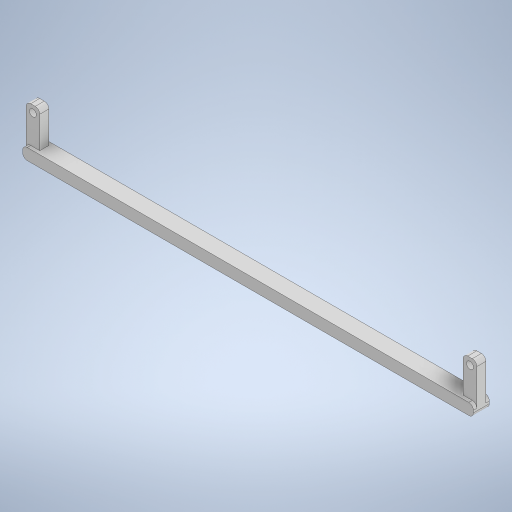
# Autodesk Inventor part: Brace_equal
Saved by Autodesk Inventor 2024.3 (Build 283343000, 343)
## iProperties
Created: 2024-11-11
Part Number: Brace_equal
Material: Generic
Document SubType Name: Modeling
Designer: magn1
Density: 1 g/cm^3
Appearance: Default
Author: magn1
Autodesk Inventor part; units mm, degrees
ref_plane "YZ Plane" through (0, 0, 0) normal (1, 0, 0) x (0, 1, 0)
ref_plane "XZ Plane" through (0, 0, 0) normal (0, 1, 0) x (-1, 0, 0)
ref_plane "XY Plane" through (0, 0, 0) normal (0, 0, 1) x (1, 0, 0)
sketch "Sketch1" plane through (0, 0, 0) normal (0, 1, 0) x (-1, 0, 0)
  line L0 (99.05, 3.5) -> (-99.05, 3.5)
  line L1 (-99.05, 3.5) -> (-99.05, -3.5)
  line L2 (-99.05, -3.5) -> (99.05, -3.5)
  line L3 (99.05, -3.5) -> (99.05, 3.5)
  line L4 (99.05, 3.5) -> (-99.05, -3.5) construction
  line L5 (-99.05, 3.5) -> (99.05, -3.5) construction
  point P0 (0, 0)
  dimension "d0" = 198.1
  dimension "d1" = 7
  constraints: 12 end point, 2 midpoint, 2 parallel, 1 horizontal, 1 perpendicular
  measures "d0" distance of L2.end L1.end
  measures "d1" distance of L1.end L0.end
extrude "Extrusion1" add sketch "Sketch1" along normal blind 5
sketch "Sketch2" plane through (0, 5, 0) normal (0, 1, 0) x (1, 0, 0)
  line L0 (-99.05, 3.5) -> (-99.05, -3.5) projected
  line L1 (-99.05, 2) -> (-93.05, 2)
  line L2 (-93.05, 2) -> (-93.05, -2)
  line L3 (-93.05, -2) -> (-99.05, -2)
  line L4 (-99.05, -2) -> (-99.05, 2)
  line L5 (99.05, 3.5) -> (-99.05, 3.5) projected
  line L6 (99.05, 2) -> (93.05, 2)
  line L7 (93.05, 2) -> (93.05, -2)
  line L8 (93.05, -2) -> (99.05, -2)
  line L9 (99.05, -2) -> (99.05, 2)
  line L10 (99.05, -3.5) -> (99.05, 3.5) projected
  point P0 (0, 0)
  dimension "d18" = 6
  dimension "d19" = 4
  dimension "d20" = 1.5
  dimension "d21" = 6
  dimension "d22" = 4
  dimension "d23" = 1.5
  dimension "d24" = 6
  constraints: 16 end point, 4 parallel, 2 horizontal, 2 perpendicular, 1 point on line
  measures "d18" distance of L2.end L3.end
  measures "d19" distance of L1.end L2.end
  measures "d20" distance between parallel lines of L5 L1
  measures "d21" distance of L8.end L7.end
  measures "d22" distance of L7.end L6.end
  measures "d23" distance between parallel lines of L5 L6
  measures "d24" distance between parallel lines of L10 L7
extrude "Extrusion2" add sketch "Sketch2" along normal blind 15.875
fillet "Fillet1" radius 2 4 edges at (-99.05, 20.875, 0) (-93.05, 20.875, 0) (99.05, 20.875, 0) (93.05, 20.875, 0)
fillet "Fillet2" radius 2 2 edges at (99.05, 0, 0) (-99.05, 0, 0)
sketch "Sketch4" plane through (-99.05, 5, 2) normal (0, 0, 1) x (1, 0, 0)
  line L0 (2, 15.875) -> (4, 15.875) construction
  line L1 (3, 15.875) -> (3, 12.875) construction
  line L2 (3, 15.875) -> (6, 15.875) construction
  circle A0 centre (3, 12.875) radius 1.5
  line L3 (196.1, 15.875) -> (194.1, 15.875) construction
  line L4 (195.1, 15.875) -> (195.1, 12.875) construction
  line L5 (195.1, 15.875) -> (198.1, 15.875) construction
  circle A1 centre (195.1, 12.875) radius 1.5
  point P0 (99.05, -5)
  dimension "d25" = 3
  dimension "d26" = 90
  dimension "d27" = 3
  dimension "d28" = 3
  dimension "d29" = 90
  dimension "d30" = 3
  constraints: 8 end point, 2 centre point, 2 coincident, 2 horizontal, 2 midpoint, 2 perpendicular, 2 vertical
  measures "d25" distance of L1.start L1.end
  measures "d26" angle of L1 L2
  measures "d27" diameter of A0
  measures "d28" distance of L4.start L4.end
  measures "d29" angle of L4 L5
  measures "d30" diameter of A1
extrude "Extrusion4" cut sketch "Sketch4" against normal through all
fillet "Fillet3" radius 2 4 edges at (-99.05, 5, 2.75) (-99.05, 5, -2.75) (99.05, 5, -2.75) (99.05, 5, 2.75)
body "Solid1"
